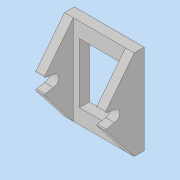
# Autodesk Inventor part: switchHolder
Saved by Autodesk Inventor 2017 (Build 210142000, 142)
## iProperties
Created: 2019-07-14
Part Number: switchHolder
Material: Generic
Document SubType Name: Modeling
Designer: techn
Density: 1 g/cm^3
Appearance: Default
Author: techn
Autodesk Inventor part; units mm, degrees
ref_plane "YZ Plane" through (0, 0, 0) normal (1, 0, 0) x (0, 1, 0)
ref_plane "XZ Plane" through (0, 0, 0) normal (0, 1, 0) x (-1, 0, 0)
ref_plane "XY Plane" through (0, 0, 0) normal (0, 0, 1) x (1, 0, 0)
sketch "Sketch1" plane through (0, 0, 0) normal (0, 0, 1) x (1, 0, 0)
  line L0 (0, 0) -> (22.225, 0)
  line L1 (22.225, 0) -> (22.225, 28.575)
  line L2 (22.225, 28.575) -> (0, 28.575)
  line L3 (0, 28.575) -> (0, 0)
  line L4 (4.7625, 4.7625) -> (17.4625, 4.7625)
  line L5 (17.4625, 4.7625) -> (17.4625, 23.8125)
  line L6 (17.4625, 23.8125) -> (4.7625, 23.8125)
  line L7 (4.7625, 23.8125) -> (4.7625, 4.7625)
  point P0 (17.4625, 14.2875)
  point P1 (22.225, 14.2875)
  point P2 (11.1125, 23.8125)
  point P3 (11.1125, 28.575)
  dimension "d0" = 22.225
  dimension "d1" = 28.575
  dimension "d2" = 19.05
  dimension "d3" = 12.7
  constraints: 16 end point, 4 midpoint, 4 parallel, 2 horizontal, 2 perpendicular, 1 horizontal alignment, 1 vertical alignment
  measures "d0" distance between parallel lines of L1 L3
  measures "d1" distance of L0.end L1.end
  measures "d2" distance of L4.end L5.end
  measures "d3" distance of L4.start L4.end
extrude "Extrusion1" add sketch "Sketch1" along normal blind 3.175
sketch "Sketch2" plane through (22.225, 0, 0) normal (1, 0, 0) x (0, 0, -1)
  line L0 (-3.175, 0) -> (-3.175, 28.575) projected
  arc A0 (-9.525, 12.5095) -> (-9.525, 16.0655) centre (-9.525, 14.2875) ccw
  arc A1 (-12.5246, 11.9383) -> (-12.5246, 16.6367) centre (-9.525, 14.2875) ccw
  line L1 (-3.175, 28.575) -> (-12.5246, 16.6367)
  line L2 (-3.175, 0) -> (-12.5246, 11.9383)
  line L3 (-12.5246, 11.9383) -> (-9.525, 12.5095)
  line L4 (-12.5246, 16.6367) -> (-9.525, 16.0655)
  point P0 (0, 0)
  point P1 (-3.175, 14.2875)
  dimension "d6" = 3.556
  dimension "d7" = 6.35
  dimension "d8" = 7.62
  constraints: 8 end point, 4 point on circle, 2 centre point, 2 tangent, 1 coincident, 1 horizontal alignment, 1 midpoint
  measures "d6" diameter of A0
  measures "d7" distance from line of L0 A0.centre
  measures "d8" diameter of A1
extrude "Extrusion2" add sketch "Sketch2" against normal blind 2.794
sketch "Sketch3" plane through (0, 0, 0) normal (-1, 0, 0) x (0, 0, 1)
  line L0 (3.175, 0) -> (3.175, 28.575) projected
  line L1 (3.175, 0) -> (12.5246, 11.9383) projected
  line L2 (12.5246, 11.9383) -> (9.525, 12.5095) projected
  arc A0 (9.525, 16.0655) -> (9.525, 12.5095) centre (9.525, 14.2875) ccw projected
  line L3 (9.525, 16.0655) -> (12.5246, 16.6367) projected
  line L4 (12.5246, 16.6367) -> (3.175, 28.575) projected
  point P0 (0, 0)
extrude "Extrusion3" add sketch "Sketch3" against normal blind 2.794
fillet "Fillet1" radius 0.254 4 edges at (1.397, 16.6367, 12.5246) (1.397, 11.9383, 12.5246) (20.828, 16.6367, 12.5246) (20.828, 11.9383, 12.5246)
body "Solid1"
